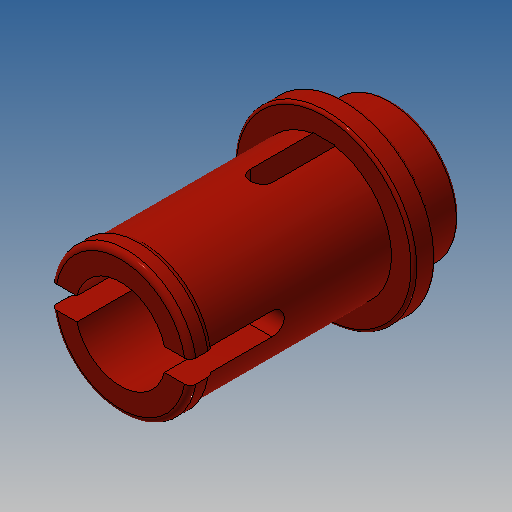
# Autodesk Inventor part: 4274-Red
Saved by Autodesk Inventor 2025 (Build 290162010, 162A)
## iProperties
Created: 2014-06-03
Part Number: 4274-Red
Material: ABS Plastic
Document SubType Name: Modeling
Designer: D. Kohfeld
Appearance: Red
Density: 1.06 g/cm^3
Mass: 0.104333 g
Surface Area: 2.93085 cm^2
Volume: 0.0984273 cm^3
Author: D. Kohfeld
Autodesk Inventor part; units mm, degrees
ref_plane "YZ Plane" through (0, 0, 0) normal (1, 0, 0) x (0, 1, 0)
ref_plane "XZ Plane" through (0, 0, 0) normal (0, 1, 0) x (-1, 0, 0)
ref_plane "XY Plane" through (0, 0, 0) normal (0, 0, 1) x (1, 0, 0)
sketch "Sketch1" plane through (0, 0, 0) normal (0, 1, 0) x (-1, 0, 0)
  line L0 (2.4, 7.2) -> (2.4, 0.8)
  line L1 (3.2, 0.8) -> (2.4, 0.8)
  line L2 (3.2, 0.8) -> (3.2, 0)
  line L3 (2.5, 8) -> (2.5, 7.2)
  line L4 (2.5, 8) -> (1.6, 8)
  line L5 (0, -3.52) -> (0, 9.92) projected
  line L6 (2.4, 7.2) -> (2.5, 7.2)
  line L7 (1.6, 8) -> (1.6, -1.6)
  line L8 (3.8, 0) -> (-1.1, 0) projected
  line L9 (-0.4, 3) -> (-0.4, 0)
  line L10 (0.4, 0) -> (0.4, 3)
  arc A0 (0.4, 3) -> (-0.4, 3) centre (0, 3) ccw
  line L11 (0.4, 0) -> (-0.4, 0)
  line L12 (1.6, -1.6) -> (2.4, -1.6)
  line L13 (2.4, -1.6) -> (2.4, 0)
  line L14 (2.4, 0) -> (3.2, 0)
  point P0 (0, 0)
  point P1 (0, 0)
  dimension "d1" = 4.8
  dimension "d2" = 5
  dimension "d6" = 8
  dimension "d7" = 0.8
  dimension "d8" = 6.4
  dimension "d9" = 0.8
  dimension "d14" = 0.8
  dimension "d32" = 3.4
  dimension "d33" = 1.6
  dimension "d36" = 0
  dimension "d37" = 3.2
  dimension "d38" = 4.8
  constraints: 24 end point, 3 parallel, 2 horizontal, 2 perpendicular, 2 point on circle, 2 tangent, 1 centre point, 1 coincident, 1 midpoint, 1 point on line, 1 vertical alignment, 3 other
  measures "d1" diameter of L0 L5
  measures "d2" diameter of L3 L5
  measures "d6" distance between parallel lines of L4 L8
  measures "d7" distance from line of L3.end L4
  measures "d8" diameter of L2 L5
  measures "d14" diameter of A0
  measures "d33" distance between parallel lines of L14 L12
  measures "d36" distance between parallel lines of L8 L14
  measures "d37" diameter of L7 L5
  measures "d38" diameter of L13 L5
revolve "Revolution1" add sketch "Sketch1" angle 360 about axis through (0, 0, -10) along (0, 0, 1) contours L0 L1 L2 L8 L7 L4 L3 L6 | L13 L12 L7 L8
fillet "Fillet1" radius 0.2 2 edges at (2.5, 0, 8) (2.5, 0, 7.2)
fillet "Fillet1" radius 0.1 3 edges at (2.4, 0, -1.6) (3.2, 0, 0) (3.2, 0, 0.8)
extrude "Extrusion1" cut sketch "Sketch1" along normal mid plane 4.8 contours L8 L9 A0 L5 | L5 A0 L10 L8
sketch "Sketch2" plane through (0, 0, 0) normal (1, 0, 0) x (0, 1, 0)
  line L0 (-1.6, 8) -> (1.6, 8) projected
  line L1 (-0.4, 8) -> (0.4, 8)
  line L2 (0.4, 8) -> (0.4, 5)
  line L3 (-0.4, 5) -> (-0.4, 8)
  arc A0 (-0.4, 5) -> (0.4, 5) centre (0, 5) ccw
  point P0 (0, 8)
  dimension "d34" = 3.4
  dimension "d35" = 0.8
  constraints: 6 end point, 2 midpoint, 2 point on circle, 2 tangent, 1 centre point, 1 horizontal, 1 parallel, 1 perpendicular, 1 point on line
  measures "d35" diameter of A0
extrude "Extrusion2" cut sketch "Sketch2" along normal through all both and the other way through all
equation "\"d1\" = tpd"
equation "\"d2\" = tpcd"
equation "\"d6\" = lu"
equation "\"d7\" = d9"
equation "\"d8\" = tsd"
equation "\"d9\" = tsl"
equation "\"d14\" = tpnw"
equation "\"d32\" = tpnl"
equation "\"d33\" = knobh"
equation "\"d37\" = rd"
equation "\"d38\" = kd"
equation "\"d27\" = pinf"
equation "\"d28\" = lf"
equation "\"d34\" = tpnl"
equation "\"d35\" = tpnw"
equation "\"tpd\" = 4.8"
equation "\"tpcd\" = 5"
equation "\"lu\" = 8"
equation "\"tsd\" = 6.4"
equation "\"tsl\" = 0.8"
equation "\"tpnw\" = 0.8"
equation "\"tpnl\" = 3.4"
equation "\"knobh\" = 1.6"
equation "\"rd\" = 3.2"
equation "\"kd\" = 4.8"
equation "\"pinf\" = 0.2"
equation "\"lf\" = 0.1"
body "Solid2"
